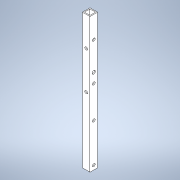
# Autodesk Inventor part: ハンド9x9_1
Saved by Autodesk Inventor 2020.3 (Build 243373000, 373)
## iProperties
Created: 2020-05-31
Part Number: ハンド9x9_1
Material: アルミニウム 6061
Document SubType Name: Modeling
Designer: totot
Mass: 14.7492 g
Surface Area: 93.5879 cm^2
Volume: 5.46268 cm^3
Density: 2.7 g/cm^3
Appearance: アルミニウム - フラット
Author: totot
Autodesk Inventor part; units mm, degrees
ref_plane "YZ Plane" through (0, 0, 0) normal (1, 0, 0) x (0, 1, 0)
ref_plane "XZ Plane" through (0, 0, 0) normal (0, 1, 0) x (-1, 0, 0)
ref_plane "XY Plane" through (0, 0, 0) normal (0, 0, 1) x (1, 0, 0)
sketch "スケッチ1" plane through (0, 0, 0) normal (0, 1, 0) x (-1, 0, 0)
  line L0 (0, 0) -> (-9, 0)
  line L1 (-9, 0) -> (-9, 9)
  line L2 (-9, 9) -> (0, 9)
  line L3 (0, 9) -> (0, 0)
  line L4 (-1.2, 7.8) -> (-7.8, 7.8)
  line L5 (-7.8, 7.8) -> (-7.8, 1.2)
  line L6 (-7.8, 1.2) -> (-1.2, 1.2)
  line L7 (-1.2, 1.2) -> (-1.2, 7.8)
  dimension "d0" = 9
  dimension "d1" = 9
  dimension "d2" = 1.2
  dimension "d3" = 1.2
  dimension "d4" = 1.2
  dimension "d5" = 1.2
  constraints: 16 end point, 4 parallel, 2 horizontal, 2 perpendicular
  measures "d0" distance of L1.end L2.end
  measures "d1" distance of L0.end L1.end
  measures "d2" distance between parallel lines of L3 L7
  measures "d3" distance between parallel lines of L2 L4
  measures "d4" distance between parallel lines of L6 L0
  measures "d5" distance between parallel lines of L1 L5
extrude "押し出し1" add sketch "スケッチ1" along normal blind 160
sketch "スケッチ2" plane through (9, 0, 9) normal (1, 0, 0) x (0, 0, -1)
  line L0 (0, 0) -> (9, 0) projected
  line L1 (0, 0) -> (0, 160) projected
  point P0 (4.5, 5)
  point P1 (4.5, 51)
  dimension "d8" = 46
  dimension "d9" = 5
  dimension "d10" = 4.5
  dimension "d11" = 4.5
  measures "d8" distance of point (4.5, 5) point (4.5, 51)
  measures "d9" distance from line of L0 point (4.5, 5)
  measures "d10" distance from line of L1 point (4.5, 51)
  measures "d11" distance from line of L1 point (4.5, 5)
hole "穴1" at (9, 5, 4.5) at (9, 51, 4.5) direction (-1, 0, 0) diameter 3.3 end through all
sketch "スケッチ3" plane through (9, 0, 9) normal (1, 0, 0) x (0, 0, -1)
  line L0 (0, 160) -> (9, 160) projected
  line L1 (9, 0) -> (9, 160) projected
  line L2 (0, 0) -> (9, 0) projected
  point P0 (4.5, 89)
  point P1 (4.5, 134)
  dimension "d20" = 4.5
  dimension "d38" = 89
  dimension "d39" = 45
  measures "d20" distance from line of L1 point (4.5, 89)
  measures "d38" distance from line of point (4.5, 89) L2
  measures "d39" distance of point (4.5, 134) point (4.5, 89)
hole "穴2" at (9, 89, 4.5) at (9, 134, 4.5) direction (-1, 0, 0) diameter 3.3 end through all
sketch "スケッチ4" plane through (0, 0, 9) normal (0, 0, 1) x (1, 0, 0)
  line L0 (0, 160) -> (9, 160) projected
  line L1 (9, 0) -> (9, 160) projected
  line L2 (0, 0) -> (9, 0) projected
  point P0 (4.5, 80)
  point P1 (4.5, 125)
  dimension "d29" = 4.5
  dimension "d37" = 80
  dimension "d40" = 45
  measures "d29" distance from line of point (4.5, 80) L1
  measures "d37" distance from line of L2 point (4.5, 80)
  measures "d40" distance of point (4.5, 80) point (4.5, 125)
hole "穴3" at (4.5, 80, 9) at (4.5, 125, 9) direction (0, 0, -1) diameter 3.3 end through all
sketch "スケッチ5" plane through (9, 0, 9) normal (1, 0, 0) x (0, 0, -1)
  line L0 (0, 0) -> (0, 160) projected
  circle A0 centre (4.5, 89) radius 1.65 projected
  point P0 (9, 0)
  point P1 (4.5, 100.5)
  dimension "d41" = 4.5
  dimension "d42" = 11.5
  measures "d41" distance from line of L0 point (4.5, 100.5)
  measures "d42" distance of A0.centre point (4.5, 100.5)
hole "穴4" at (9, 100.5, 4.5) direction (-1, 0, 0) diameter 4 end through all
equation "\"d3\" = d2"
equation "\"d4\" = d2"
equation "\"d5\" = d3"
